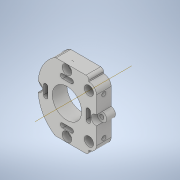
# Autodesk Inventor part: 20_Cube_Insert_Kinematic_VCAmount_Base_Thorlabs_Cage_smaller
Saved by Autodesk Inventor 2022.3 (Build 263350000, 350)
## iProperties
Created: 2019-07-01
Part Number: 20_Cube_Insert_Kinematic_VCAmount_Base_Thorlabs_Cage_smaller
Material: Generic
Document SubType Name: Modeling
Designer: diederichbenedict
Density: 1 g/cm^3
Appearance: Default
Author: diederichbenedict
Autodesk Inventor part; units mm, degrees
ref_plane "YZ Plane" through (0, 0, 0) normal (1, 0, 0) x (0, 1, 0)
ref_plane "Work Plane1" through (0, 0, 10) normal (0, 0, 1) x (1, 0, 0)
sketch "Sketch1" plane through (0, 0, 10) normal (0, 0, 1) x (1, 0, 0)
  line L0 (-4.0299, -0.3538) -> (-2.2322, 1.4439) construction
  arc A0 (-1.4439, 2.2322) -> (-2.2322, 1.4439) centre (-0.9299, 0.9299) ccw construction
  line L1 (-1.4439, 2.2322) -> (0.3538, 4.0299) construction
  line L2 (-37.8299, 42.8299) -> (-37.8299, 37.8299) construction
  line L3 (-37.8299, 37.8299) -> (-42.9208, 37.8299) construction
  line L4 (-37.8299, 42.2137) -> (-37.8299, 45.8299) construction
  line L5 (-37.8299, 45.8299) -> (-4.0299, 45.8299) construction
  line L6 (-4.0299, 45.8299) -> (-4.0299, 42.2137) construction
  line L7 (-4.0299, 4.0299) -> (0.3538, 4.0299) projected
  circle A1 centre (-20.9299, 20.9299) radius 17.5 projected
  line L8 (-20.9299, 58.9723) -> (17.1124, 20.9299) construction
  line L9 (17.1124, 20.9299) -> (-20.9299, -17.1124) construction
  line L10 (-20.9299, -17.1124) -> (-58.9723, 20.9299) construction
  line L11 (-58.9723, 20.9299) -> (-20.9299, 58.9723) construction
  line L12 (-20.9299, 58.9723) -> (-20.9299, -17.1124) construction
  line L13 (17.1124, 20.9299) -> (-58.9723, 20.9299) construction
  line L14 (-20.9299, 58.9723) -> (32.8701, 58.9723) construction
  line L15 (-43.4299, 43.4299) -> (1.5701, 43.4299) construction
  line L16 (1.5701, 43.4299) -> (1.5701, -1.5701) construction
  line L17 (1.5701, -1.5701) -> (-43.4299, -1.5701) construction
  line L18 (-43.4299, -1.5701) -> (-43.4299, 43.4299) construction
  line L19 (-43.4299, 43.4299) -> (1.5701, -1.5701) construction
  line L20 (1.5701, 43.4299) -> (-43.4299, -1.5701) construction
  line L21 (-43.4299, 5.3876) -> (-43.4299, 36.4723)
  line L22 (-43.4299, 36.4723) -> (-36.4723, 43.4299)
  line L23 (-36.4723, 43.4299) -> (-5.3876, 43.4299)
  line L24 (-5.3876, 43.4299) -> (1.5701, 36.4723)
  line L25 (1.5701, 36.4723) -> (1.5701, 5.3876)
  line L26 (1.5701, 5.3876) -> (-5.3876, -1.5701)
  line L27 (-5.3876, -1.5701) -> (-36.4723, -1.5701)
  line L28 (-36.4723, -1.5701) -> (-43.4299, 5.3876)
  line L29 (-4.0299, 42.2137) -> (-37.8299, 42.2137) projected
  line L30 (-4.0299, -0.3538) -> (-4.0299, 4.0299) projected
  point P0 (-37.8299, 4.0299)
  point P1 (-20.9299, 20.9299)
  dimension "d18" = 53.8
  dimension "d19" = 45
  dimension "d20" = 53.8
  dimension "d21" = 45
  dimension "d22" = 45
  constraints: 42 end point, 15 point on line, 5 midpoint, 4 parallel, 3 perpendicular, 2 horizontal, 1 equal length
  measures "d18" distance of L8.start L8.end
  measures "d19" angle of L8 L14
  measures "d20" distance of L8.end L9.end
  measures "d21" distance of L16.end L17.end
  measures "d22" distance of L15.end L16.end
extrude "Extrusion1" add sketch "Sketch1" along normal blind 10 contours L30 L26 L27 L28 L21 L22 L29 L24 L25 L7 | L7 L26 L30 | L29 L22 L23 L24 | A1
ref_plane "Work Plane2" through (-40.9959, 0.8639, 22.2359) normal (0, 0, 1) x (1, 0, 0)
sketch "Sketch3" plane through (0, 0, 10) normal (0, 0, -1) x (-1, 0, 0)
  line L0 (37.8299, -0.4701) -> (37.8299, 4.0299) construction
  line L1 (4.0299, 4.0299) -> (4.0299, -0.4701) construction
  line L2 (37.8299, -0.4701) -> (37.8299, 1.1886) construction
  line L3 (4.0299, -3.9701) -> (4.0299, -0.3538) construction
  line L4 (45.8299, 4.0299) -> (42.2137, 4.0299) construction
  line L5 (-0.3538, 4.0299) -> (-3.9701, 4.0299) construction
  line L6 (-3.9701, 37.8299) -> (-0.3538, 37.8299) construction
  line L7 (4.0299, 42.2137) -> (4.0299, 45.8299) construction
  line L8 (37.8299, 45.8299) -> (37.8299, 42.2137) construction
  line L9 (42.2137, 37.8299) -> (45.8299, 37.8299) construction
  line L10 (40.4657, 37.7299) -> (45.8299, 37.7299)
  line L11 (45.8299, 37.7299) -> (45.8299, 4.1299)
  line L12 (45.8299, 4.1299) -> (40.4657, 4.1299)
  line L13 (40.4657, 4.1299) -> (40.4657, 37.7299)
  line L14 (37.7299, 2.4952) -> (4.1299, 2.4952)
  line L15 (4.1299, 2.4952) -> (4.1299, -3.9701)
  line L16 (4.1299, -3.9701) -> (37.7299, -3.9701)
  line L17 (37.7299, -3.9701) -> (37.7299, 2.4952)
  line L18 (1.8946, 4.1299) -> (-3.9701, 4.1299)
  line L19 (-3.9701, 4.1299) -> (-3.9701, 37.7299)
  line L20 (-3.9701, 37.7299) -> (1.8946, 37.7299)
  line L21 (1.8946, 37.7299) -> (1.8946, 4.1299)
  line L22 (4.1299, 40.7326) -> (37.7299, 40.7326)
  line L23 (37.7299, 40.7326) -> (37.7299, 45.8299)
  line L24 (37.7299, 45.8299) -> (4.1299, 45.8299)
  line L25 (4.1299, 45.8299) -> (4.1299, 40.7326)
  point P0 (0, 0)
  dimension "d23" = 0.1
  dimension "d24" = 0.1
  dimension "d25" = 0.1
  dimension "d26" = 0.1
  dimension "d27" = 0.1
  constraints: 32 end point, 8 parallel, 4 horizontal, 4 perpendicular, 3 point on line
  measures "d23" distance between parallel lines of L8 L23
  measures "d24" distance between parallel lines of L7 L25
  measures "d25" distance between parallel lines of L6 L20
  measures "d26" distance between parallel lines of L5 L18
  measures "d27" distance between parallel lines of L1 L15
extrude "Extrusion3" add sketch "Sketch3" against normal up to surface (10 mm away)
sketch "Sketch4" plane through (0, 0, 20) normal (0, 0, 1) x (1, 0, 0)
  line L0 (3.9701, 4.1299) -> (0.3124, 4.1299) projected
  line L1 (3.9701, 37.7299) -> (3.9701, 4.1299) projected
  line L2 (0.3124, 37.7299) -> (3.9701, 37.7299) projected
  line L3 (0.3124, 37.7299) -> (-4.1299, 42.1723) projected
  line L4 (-4.1299, 45.8299) -> (-4.1299, 42.1723) projected
  line L5 (-37.7299, 45.8299) -> (-4.1299, 45.8299) projected
  line L6 (-37.7299, 42.1723) -> (-37.7299, 45.8299) projected
  line L7 (-37.7299, 42.1723) -> (-42.1723, 37.7299) projected
  line L8 (-45.8299, 37.7299) -> (-42.1723, 37.7299) projected
  line L9 (-45.8299, 4.1299) -> (-45.8299, 37.7299) projected
  line L10 (-42.1723, 4.1299) -> (-45.8299, 4.1299) projected
  line L11 (-42.1723, 4.1299) -> (-37.7299, -0.3124) projected
  line L12 (-37.7299, -3.9701) -> (-37.7299, -0.3124) projected
  line L13 (-4.1299, -3.9701) -> (-37.7299, -3.9701) projected
  line L14 (-4.1299, -0.3124) -> (-4.1299, -3.9701) projected
  line L15 (-4.1299, -0.3124) -> (0.3124, 4.1299) projected
  line L16 (-3.9799, 45.9799) -> (-3.9799, 42.2344)
  line L17 (-3.9799, 42.2344) -> (0.3745, 37.8799)
  line L18 (0.3745, 37.8799) -> (4.1201, 37.8799)
  line L19 (4.1201, 37.8799) -> (4.1201, 3.9799)
  line L20 (4.1201, 3.9799) -> (0.3745, 3.9799)
  line L21 (0.3745, 3.9799) -> (-3.9799, -0.3745)
  line L22 (-3.9799, -0.3745) -> (-3.9799, -4.1201)
  line L23 (-3.9799, -4.1201) -> (-37.8799, -4.1201)
  line L24 (-37.8799, -4.1201) -> (-37.8799, -0.3745)
  line L25 (-37.8799, -0.3745) -> (-42.2344, 3.9799)
  line L26 (-42.2344, 3.9799) -> (-45.9799, 3.9799)
  line L27 (-45.9799, 3.9799) -> (-45.9799, 37.8799)
  line L28 (-45.9799, 37.8799) -> (-42.2344, 37.8799)
  line L29 (-42.2344, 37.8799) -> (-37.8799, 42.2344)
  line L30 (-37.8799, 42.2344) -> (-37.8799, 45.9799)
  line L31 (-37.8799, 45.9799) -> (-3.9799, 45.9799)
  point P0 (0, 0)
  dimension "d34" = 0.15
  constraints: 32 end point, 15 other
  measures "d34" distance between parallel lines of L5 L31
extrude "Extrusion4" add sketch "Sketch4" against normal up to surface (10 mm away)
sketch "Sketch8" plane through (0, 0, 20) normal (0, 0, 1) x (1, 0, 0)
  circle A0 centre (-20.9299, 20.9299) radius 10
  line L0 (4.1201, 37.8799) -> (4.1201, 3.9799) projected
  line L1 (-37.8799, 45.9799) -> (-3.9799, 45.9799) projected
  point P0 (0, 0)
  point P1 (4.1201, 20.9299)
  point P2 (-20.9299, 45.9799)
  dimension "d61" = 20
  constraints: 2 midpoint, 1 centre point, 1 horizontal alignment, 1 vertical alignment
  measures "d61" diameter of A0
ref_plane "Work Plane3" through (-40.0572, 1.8027, 20) normal (-0.7071, 0.7071, 0) x (0.7071, 0.7071, 0)
sketch "Sketch5" plane through (0, 0, 20) normal (0, 0, 1) x (1, 0, 0)
  circle A0 centre (-20.9299, 20.9299) radius 29.7458 construction
  line L0 (4.1201, 37.8799) -> (4.1201, 3.9799) projected
  line L1 (-37.8799, 45.9799) -> (-3.9799, 45.9799) projected
  line L2 (-34.9299, 6.9299) -> (-6.9299, 6.9299) construction
  line L3 (-6.9299, 6.9299) -> (-6.9299, 34.9299) construction
  line L4 (-6.9299, 34.9299) -> (-34.9299, 34.9299) construction
  line L5 (-34.9299, 34.9299) -> (-34.9299, 6.9299) construction
  line L6 (-34.9299, 6.9299) -> (-6.9299, 34.9299) construction
  line L7 (-6.9299, 6.9299) -> (-34.9299, 34.9299) construction
  line L8 (-40.7289, 20.9299) -> (-20.9299, 40.7289)
  line L9 (-20.9299, 40.7289) -> (-1.1309, 20.9299)
  line L10 (-1.1309, 20.9299) -> (-20.9299, 1.1309)
  line L11 (-20.9299, 1.1309) -> (-40.7289, 20.9299)
  line L12 (-40.7289, 20.9299) -> (-1.1309, 20.9299) construction
  line L13 (-20.9299, 40.7289) -> (-20.9299, 1.1309) construction
  line L14 (-3.9799, -4.1201) -> (-37.8799, -4.1201) construction
  point P0 (0, 0)
  point P1 (4.1201, 20.9299)
  point P2 (-20.9299, 45.9799)
  point P3 (0, 0)
  point P4 (-20.9299, 20.9299)
  point P5 (-20.9299, 20.9299)
  point P6 (-20.9299, 45.9799)
  point P7 (-20.9299, -4.1201)
  point P8 (4.1201, 20.9299)
  dimension "d37" = 28
  dimension "d38" = 28
  dimension "d41" = 28
  dimension "d42" = 28
  constraints: 24 end point, 8 midpoint, 4 coincident, 4 parallel, 3 vertical alignment, 2 horizontal alignment, 2 perpendicular, 1 centre point, 1 horizontal
  measures "d37" distance of L4.end L3.end
  measures "d38" distance of L3.end L2.end
  measures "d41" distance of L10.end L8.start
  measures "d42" distance of L8.start L8.end
hole "Hole1" at (-20.9299, 40.7289, 20) at (-1.1309, 20.9299, 20) at (-20.9299, 1.1309, 20) at (-40.7289, 20.9299, 20) direction (0, 0, -1) diameter 2.85 end through all counterbore diameter 6.5 counterbore depth 4
sketch "Sketch6" plane through (0, 0, 20) normal (0, 0, 1) x (1, 0, 0)
  circle A0 centre (-1.1311, 20.9299) radius 3.25
  line L0 (-17.9299, 6.3799) -> (-23.9299, 6.3799) construction
  line L1 (-17.9299, 7.8799) -> (-23.9299, 7.8799)
  line L2 (-23.9299, 4.8799) -> (-17.9299, 4.8799)
  arc A1 (-17.9299, 4.8799) -> (-16.4299, 6.3799) centre (-17.9299, 6.3799) ccw
  arc A2 (-23.9299, 7.8799) -> (-25.4299, 6.3799) centre (-23.9299, 6.3799) ccw
  circle A3 centre (-20.9299, 40.7289) radius 3.25 projected
  line L3 (-3.9799, 45.9799) -> (-3.9799, 42.2344) projected
  line L4 (-37.8799, 45.9799) -> (-3.9799, 45.9799) projected
  line L5 (-37.8799, 42.2344) -> (-37.8799, 45.9799) projected
  line L6 (-42.2344, 37.8799) -> (-37.8799, 42.2344) projected
  line L7 (-45.9799, 37.8799) -> (-42.2344, 37.8799) projected
  line L8 (-45.9799, 3.9799) -> (-45.9799, 37.8799) projected
  line L9 (-42.2344, 3.9799) -> (-45.9799, 3.9799) projected
  line L10 (-37.8799, -0.3745) -> (-42.2344, 3.9799) projected
  line L11 (-37.8799, -4.1201) -> (-37.8799, -0.3745) projected
  line L12 (-3.9799, -4.1201) -> (-37.8799, -4.1201) projected
  line L13 (-3.9799, -0.3745) -> (-3.9799, -4.1201) projected
  line L14 (0.3745, 3.9799) -> (-3.9799, -0.3745) projected
  line L15 (4.1201, 3.9799) -> (0.3745, 3.9799) projected
  line L16 (4.1201, 37.8799) -> (4.1201, 3.9799) projected
  line L17 (0.3745, 37.8799) -> (4.1201, 37.8799) projected
  line L18 (-3.9799, 42.2344) -> (0.3745, 37.8799) projected
  circle A4 centre (-20.9299, 40.7289) radius 3.25 projected
  line L19 (-3.9799, 45.9799) -> (-3.9799, 42.2344) projected
  line L20 (-37.8799, 45.9799) -> (-3.9799, 45.9799) projected
  line L21 (-37.8799, 42.2344) -> (-37.8799, 45.9799) projected
  line L22 (-42.2344, 37.8799) -> (-37.8799, 42.2344) projected
  line L23 (-45.9799, 37.8799) -> (-42.2344, 37.8799) projected
  line L24 (-45.9799, 3.9799) -> (-45.9799, 37.8799) projected
  line L25 (-42.2344, 3.9799) -> (-45.9799, 3.9799) projected
  line L26 (-37.8799, -0.3745) -> (-42.2344, 3.9799) projected
  line L27 (-37.8799, -4.1201) -> (-37.8799, -0.3745) projected
  line L28 (-3.9799, -4.1201) -> (-37.8799, -4.1201) projected
  line L29 (-3.9799, -0.3745) -> (-3.9799, -4.1201) projected
  line L30 (0.3745, 3.9799) -> (-3.9799, -0.3745) projected
  line L31 (4.1201, 3.9799) -> (0.3745, 3.9799) projected
  line L32 (4.1201, 37.8799) -> (4.1201, 3.9799) projected
  line L33 (0.3745, 37.8799) -> (4.1201, 37.8799) projected
  line L34 (-3.9799, 42.2344) -> (0.3745, 37.8799) projected
  line L35 (-23.9299, 33.9799) -> (-17.9299, 33.9799)
  arc A5 (-23.9299, 36.9799) -> (-25.4299, 35.4799) centre (-23.9299, 35.4799) ccw
  arc A6 (-17.9299, 33.9799) -> (-16.4299, 35.4799) centre (-17.9299, 35.4799) ccw
  line L36 (-17.9299, 36.9799) -> (-23.9299, 36.9799)
  line L37 (-17.9299, 35.4799) -> (-23.9299, 35.4799) construction
  arc A7 (-7.8799, 17.9341) -> (-6.3799, 16.4341) centre (-6.3799, 17.9341) ccw
  line L38 (-7.8799, 23.9299) -> (-7.8799, 17.9341)
  line L39 (-6.3799, 17.9341) -> (-6.3799, 22.4299) construction
  line L40 (-4.8799, 17.9341) -> (-4.8799, 23.9299)
  circle A8 centre (-20.9299, 40.7289) radius 3.25
  arc A9 (-4.8799, 23.9299) -> (-6.3799, 25.4299) centre (-6.3799, 23.9299) ccw
  line L41 (-45.9799, 3.9799) -> (-45.9799, 37.8799) projected
  circle A10 centre (-40.7289, 20.9299) radius 3.25 projected
  circle A11 centre (-40.7289, 20.9299) radius 1.425 projected
  line L42 (4.1201, 37.8799) -> (4.1201, 3.9799) projected
  circle A12 centre (-20.9299, 1.1309) radius 3.25 projected
  circle A13 centre (-20.9299, 1.1309) radius 1.425 projected
  line L43 (-37.8799, 45.9799) -> (-3.9799, 45.9799) projected
  line L44 (-3.9799, -4.1201) -> (-37.8799, -4.1201) projected
  arc A14 (-6.3799, 16.4341) -> (-4.8799, 17.9341) centre (-6.3799, 17.9341) ccw
  arc A15 (-6.3799, 25.4299) -> (-7.8799, 23.9299) centre (-6.3799, 23.9299) ccw
  line L45 (-6.3799, 22.4299) -> (-6.3799, 23.9299) construction
  arc A16 (-16.4299, 35.4799) -> (-17.9299, 36.9799) centre (-17.9299, 35.4799) ccw
  arc A17 (-25.4299, 35.4799) -> (-23.9299, 33.9799) centre (-23.9299, 35.4799) ccw
  arc A18 (-16.4299, 6.3799) -> (-17.9299, 7.8799) centre (-17.9299, 6.3799) ccw
  arc A19 (-25.4299, 6.3799) -> (-23.9299, 4.8799) centre (-23.9299, 6.3799) ccw
  circle A20 centre (-40.7289, 20.9299) radius 3.25
  arc A21 (-36.8215, 17.9341) -> (-35.3215, 16.4341) centre (-35.3215, 17.9341) ccw
  line L46 (-36.8215, 23.9257) -> (-36.8215, 17.9341)
  line L47 (-35.3215, 23.9257) -> (-35.3215, 19.4341) construction
  line L48 (-33.8215, 17.9341) -> (-33.8215, 23.9257)
  arc A22 (-33.8215, 23.9257) -> (-35.3215, 25.4257) centre (-35.3215, 23.9257) ccw
  arc A23 (-35.3215, 25.4257) -> (-36.8215, 23.9257) centre (-35.3215, 23.9257) ccw
  arc A24 (-35.3215, 16.4341) -> (-33.8215, 17.9341) centre (-35.3215, 17.9341) ccw
  line L49 (-35.3215, 19.4341) -> (-35.3215, 17.9341) construction
  point P0 (-20.9299, 6.3799)
  point P1 (-20.9299, 20.9299)
  point P2 (-20.9299, 45.9799)
  point P3 (-45.9799, 20.9299)
  point P4 (4.1201, 20.9299)
  point P5 (-40.7289, 40.7289)
  point P6 (-20.9299, 35.4799)
  point P7 (66.7709, 47.2309)
  point P8 (-45.9801, 20.9299)
  point P9 (-1.8027, 1.8027)
  point P10 (-20.9299, 7.8799)
  point P11 (-6.3799, 20.9299)
  point P12 (-20.9299, 45.9802)
  point P13 (-40.0572, 40.0572)
  point P14 (-20.9299, 36.9799)
  point P15 (-1.8027, 40.0572)
  point P16 (-4.8799, 20.932)
  point P17 (-1.8027, 40.0572)
  point P18 (-45.9801, 20.9299)
  point P19 (-40.0573, 1.8027)
  point P20 (-40.0573, 1.8027)
  point P21 (-20.9299, 45.9799)
  point P22 (4.1201, 20.9299)
  point P23 (4.1201, 20.9299)
  point P24 (-20.9299, -4.1201)
  point P25 (-35.4799, 20.9299)
  point P26 (-36.8215, 20.9299)
  dimension "d52" = 3
  dimension "d53" = 3
  dimension "d87" = 3
  dimension "d88" = 3
  dimension "d91" = 3
  dimension "d92" = 3
  dimension "d130" = 10.5
  dimension "d131" = 10.5
  dimension "d132" = 10.5
  dimension "d159" = 3
  dimension "d160" = 3
  dimension "d161" = 10.5
  dimension "d162" = 5.2489
  dimension "d163" = 5.249
  constraints: 34 end point, 34 point on circle, 32 tangent, 19 centre point, 17 midpoint, 10 point on line, 8 horizontal alignment, 8 parallel, 4 vertical alignment, 1 coincident
  measures "d52" distance of point (-20.93, 6.38) L0.end
  measures "d53" diameter of A2
  measures "d87" distance of point (-20.93, 35.48) L37.end
  measures "d88" diameter of A5
  measures "d91" distance of point (-6.38, 20.93) L45.end
  measures "d92" diameter of A9
  measures "d130" distance from line of L4 point (-20.93, 35.48)
  measures "d131" distance from line of L16 point (-6.38, 20.93)
  measures "d132" distance from line of L12 point (-20.93, 6.38)
  measures "d159" distance of point (-35.48, 20.93) L49.end
  measures "d160" diameter of A21
  measures "d161" distance from line of L8 point (-35.48, 20.93)
  measures "d162" distance of A0.centre point (-6.38, 20.93)
  measures "d163" distance of point (-35.48, 20.93) A10.centre
extrude "Extrusion5" cut sketch "Sketch6" against normal through all contours A18 A1 L2 A19 A2 L1 | A17 A5 L36 A16 A6 L35 | L38 A15 A9 L40 A14 A7 | L46 A23 A22 L48 A24 A21
extrude "Extrusion6" cut sketch "Sketch8" against normal through all
sketch "Sketch2" plane through (0, 0, 20) normal (0, 0, 1) x (1, 0, 0)
  circle A0 centre (-35.9299, 35.9299) radius 3.0099 construction
  circle A1 centre (-5.93, 35.9299) radius 3.0099 construction
  circle A2 centre (-5.93, 5.93) radius 3.0099 construction
  circle A3 centre (-35.9299, 5.93) radius 3.0099 construction
  circle A4 centre (-35.9299, 35.9299) radius 3.125 construction
  circle A5 centre (-5.93, 35.9299) radius 3.125 construction
  circle A6 centre (-5.93, 5.93) radius 3.125 construction
  circle A7 centre (-35.9299, 5.93) radius 3.125 construction
  line L0 (1.5701, 5.3876) -> (1.5701, 36.4723) projected
  line L1 (-5.3876, 43.4299) -> (-36.4723, 43.4299) projected
  line L2 (-36.4723, 43.4299) -> (-43.4299, 36.4723) projected
  line L3 (-4.8799, 23.9299) -> (-4.8799, 17.9341) projected
  line L4 (-23.9299, 7.8799) -> (-17.9299, 7.8799) projected
  line L5 (-23.9299, 36.9799) -> (-17.9299, 36.9799) projected
  circle A8 centre (-5.93, 5.93) radius 5.1
  circle A9 centre (-5.93, 35.9299) radius 5.1
  point P0 (0, 0)
  point P1 (-20.9299, 20.9299)
  point P2 (1.5701, 20.9299)
  point P3 (-20.9299, 43.4299)
  point P4 (-35.9299, 35.9299)
  point P5 (-38.1396, 38.1396)
  point P6 (-36.7387, 32.9114)
  point P7 (-32.9114, 36.7387)
  point P8 (-5.1211, 32.9114)
  point P9 (-4.0799, 33.1904)
  point P10 (-4.1189, 8.6799)
  point P11 (-9.902, 8.6799)
  dimension "d31" = 6.25
  dimension "d32" = 6.25
  dimension "d33" = 6.25
  dimension "d102" = 6.25
  dimension "d110" = 0.2412
  dimension "d140" = 10.2
  dimension "d141" = 10.2
  constraints: 6 centre point, 3 point on circle, 2 midpoint, 1 coincident, 1 horizontal alignment, 1 vertical alignment
  measures "d31" diameter of A5
  measures "d32" diameter of A6
  measures "d33" diameter of A7
  measures "d102" diameter of A4
  measures "d110" distance from line of L3 point (-5.121, 32.911)
  measures "d140" diameter of A8
  measures "d141" diameter of A9
sketch "Sketch9" plane through (4.1201, 3.9799, 20) normal (1, 0, 0) x (0, 0, -1)
  line L0 (0, 0) -> (10, 0) projected
  line L1 (0, 33.9) -> (10, 33.9) projected
  point P0 (20, -3.9799)
  point P1 (5, 4)
  point P2 (5, 0)
  point P3 (5, 29.9)
  point P4 (5, 33.9)
  dimension "d64" = 4
  dimension "d65" = 4
  constraints: 2 midpoint, 2 vertical alignment
  measures "d64" distance from line of L0 point (5, 4)
  measures "d65" distance from line of L1 point (5, 29.9)
hole "Hole2" at (4.1201, 7.9799, 15) at (4.1201, 33.8799, 15) direction (-1, 0, 0) diameter 2.9 depth 10 tip angle 118
extrude "Extrusion7" [suppressed]
sketch "Sketch10" plane through (0, 0, 20) normal (0, 0, 1) x (1, 0, 0)
  line L0 (-37.8799, 45.9799) -> (-3.9799, 45.9799) projected
  line L1 (-36.4799, 45.9799) -> (-37.0382, 45.9799)
  line L2 (-42.2344, 3.9799) -> (-45.9799, 3.9799) projected
  line L3 (-45.9799, 3.9799) -> (-42.2344, 3.9799)
  line L4 (-3.9799, 45.9799) -> (-3.9799, 42.2344) projected
  line L5 (-3.9799, 43.9799) -> (-5.9799, 43.9799)
  line L6 (-36.4799, 45.9799) -> (-34.1344, 45.9799)
  line L7 (-3.9799, 43.9799) -> (-3.9799, 45.9799)
  line L8 (-3.9799, -4.1201) -> (-3.9799, -2.1201)
  line L9 (-3.9799, -0.3745) -> (-3.9799, -4.1201) projected
  line L10 (-3.9799, -2.1201) -> (-5.7255, -2.1201)
  line L11 (-34.1344, 45.9799) -> (-28.9151, 45.9799)
  circle A0 centre (-5.93, 5.93) radius 3.0099 projected
  circle A1 centre (-5.93, 35.9299) radius 3.0099 projected
  arc A2 (-0.83, 5.93) -> (-5.9799, 0.8302) centre (-5.93, 5.93) ccw
  arc A3 (-3.9799, 40.6424) -> (-5.9799, 41.0297) centre (-5.93, 35.9299) ccw
  line L12 (-3.9799, 43.9799) -> (-3.9799, 40.6424)
  line L13 (-0.83, 35.9299) -> (-0.83, 24.166)
  line L14 (-3.9799, -0.3745) -> (-3.9799, 1.2175)
  line L15 (-5.9799, -2.171) -> (-5.9799, 0.8302)
  line L16 (-5.9799, 41.0297) -> (-5.9799, 43.9799)
  circle A4 centre (-1.1309, 20.9299) radius 3.25 projected
  circle A5 centre (-1.1309, 20.9299) radius 1.425 projected
  circle A6 centre (-1.1309, 20.9299) radius 3.25 projected
  line L17 (-3.9799, -4.1201) -> (-0.83, -4.1201)
  line L18 (6.2025, -4.1201) -> (6.2025, 45.9799)
  line L19 (6.2025, 45.9799) -> (4.1201, 45.9799)
  circle A7 centre (-5.93, 5.93) radius 3.1599
  circle A8 centre (-5.93, 35.9299) radius 3.1599
  arc A9 (-3.9799, 1.2175) -> (-1.2175, 3.9799) centre (-5.93, 5.93) ccw
  arc A10 (-1.2175, 3.9799) -> (-0.83, 5.93) centre (-5.93, 5.93) ccw
  line L20 (-0.83, 17.6939) -> (-0.83, 5.93)
  line L21 (-0.83, 24.166) -> (-0.83, 17.6939)
  arc A11 (-0.83, 35.9299) -> (-1.2175, 37.8799) centre (-5.93, 35.9299) ccw
  arc A12 (-5.9799, 41.0297) -> (-10.6424, 37.8799) centre (-5.93, 35.9299) ccw
  line L22 (0.3745, 3.9799) -> (-3.9799, -0.3745) projected
  line L23 (-3.9799, -0.3745) -> (-3.9799, -2.1201)
  line L24 (-3.9799, 1.2175) -> (-3.9799, -0.3745)
  line L25 (-5.9799, 41.0297) -> (-5.9799, 43.9799)
  line L26 (-3.9799, 43.9799) -> (-3.9799, 40.6424)
  line L27 (-3.9799, -0.3745) -> (-3.9799, -2.1201)
  arc A13 (-5.9799, 0.8302) -> (-3.9799, 1.2175) centre (-5.93, 5.93) ccw
  line L28 (-5.7255, -2.1201) -> (-5.9799, -2.171)
  arc A14 (-10.6424, 37.8799) -> (-0.83, 35.9299) centre (-5.93, 35.9299) ccw
  arc A15 (-1.2175, 37.8799) -> (-3.9799, 40.6424) centre (-5.93, 35.9299) ccw
  line L29 (-0.83, 45.9799) -> (-3.9799, 45.9799)
  line L30 (-5.9799, 45.9799) -> (-3.9799, 45.9799)
  line L31 (-28.9151, 45.9799) -> (-5.9799, 45.9799)
  line L32 (-37.0382, 45.9799) -> (-37.8799, 45.9799)
  line L33 (-5.9799, -4.1201) -> (-3.9799, -4.1201)
  line L34 (4.1201, 37.8799) -> (4.1201, 3.9799) projected
  line L35 (-3.9799, -4.1201) -> (-37.8799, -4.1201) projected
  line L36 (-5.9799, -4.1201) -> (-7.7255, -4.1201)
  line L37 (-37.8799, -0.3745) -> (-42.2344, 3.9799) projected
  line L38 (-37.8799, -4.1201) -> (-37.8799, -2.1201)
  line L39 (-37.8799, -0.3745) -> (-42.2344, 3.9799)
  line L40 (-42.2344, 3.9799) -> (-45.9799, 3.9799)
  line L41 (-45.9799, 3.9799) -> (-45.9799, 37.8799) projected
  line L42 (-45.9799, 3.9799) -> (-45.9799, 7.7255)
  line L43 (-42.2344, 37.8799) -> (-37.8799, 42.2344) projected
  line L44 (-45.9799, 37.8799) -> (-42.2344, 37.8799)
  line L45 (-42.2344, 37.8799) -> (-37.8799, 42.2344)
  line L46 (-37.8799, 45.9799) -> (-3.9799, 45.9799) projected
  line L47 (-37.8799, 42.2344) -> (-37.8799, 43.9799)
  line L48 (-37.8799, 43.9799) -> (-37.8799, 45.9799)
  line L49 (-45.9799, 34.1344) -> (-45.9799, 37.8799)
  line L50 (-45.9799, 7.7255) -> (-45.9799, 34.1344)
  line L51 (-37.8799, -2.1201) -> (-37.8799, -0.3745)
  line L52 (-34.1344, -4.1201) -> (-37.8799, -4.1201)
  line L53 (-7.7255, -4.1201) -> (-25.1869, -4.1201)
  line L54 (-0.83, -4.1201) -> (6.2025, -4.1201)
  line L55 (4.1201, 45.9799) -> (-0.83, 45.9799)
  line L56 (-5.9799, 43.9799) -> (-28.9151, 43.9799)
  line L57 (-5.9799, -2.171) -> (-28.9151, -2.171)
  circle A16 centre (-40.7289, 20.9299) radius 3.25 projected
  line L58 (-40.4789, 17.6896) -> (-40.4789, 24.1703)
  arc A17 (-40.4789, 17.6896) -> (-37.8799, 7.7697) centre (-15.5098, 18.931) ccw
  arc A18 (-28.9151, 43.9799) -> (-35.5096, 37.8799) centre (-15.5124, 22.8762) ccw
  arc A19 (-37.8799, 7.7697) -> (-35.5463, 3.9799) centre (-15.5098, 18.931) ccw
  arc A20 (-37.8799, 34.0429) -> (-40.4789, 24.1703) centre (-15.5124, 22.8762) ccw
  arc A21 (-28.995, -2.1201) -> (-28.9151, -2.171) centre (-15.5098, 18.931) ccw
  arc A22 (-35.5463, 3.9799) -> (-28.995, -2.1201) centre (-15.5098, 18.931) ccw
  arc A23 (-35.5096, 37.8799) -> (-37.8799, 34.0429) centre (-15.5124, 22.8762) ccw
  line L59 (-25.1869, -4.1201) -> (-34.1344, -4.1201)
  point P0 (0, 0)
  point P1 (-0.83, 24.166)
  dimension "d127" = 2
  dimension "d137" = 10.2
  dimension "d138" = 10.2
  dimension "d139" = 2
  dimension "d142" = 0.15
  dimension "d143" = 0.15
  dimension "d147" = 6.0198
  dimension "d155" = 46.151
  dimension "d157" = 25
  dimension "d158" = 25
  constraints: 99 end point, 37 point on circle, 24 point on line, 18 centre point, 15 perpendicular, 13 collinear, 12 parallel, 10 horizontal, 6 tangent, 4 vertical, 1 coincident
  measures "d127" distance between parallel lines of L0 L5
  measures "d137" diameter of A2
  measures "d138" diameter of A3
  measures "d139" distance between parallel lines of L15 L9
  measures "d142" radial gap between concentric circles of A0 A7
  measures "d143" radial gap between concentric circles of A1 A8
  measures "d147" diameter of A1
  measures "d155" distance between parallel lines of L56 L57
  measures "d157" radius of A17
  measures "d158" radius of A18
extrude "Extrusion8" cut sketch "Sketch10" against normal through all contours L0 L4 L5 L56 A18 A23 A20 A16 A17 A19 A22 A21 L57 L28 L10 L8 L33 L35 L38 L51 L37 L2 L41 L44 L43 L47 L48 | L29 L55 L19 L18 L54 L17 L8 L9 L14 A9 A10 L20 A4 L13 A11 A15 L12 L4 | L4 L12 A3 L16 L5 | L10 L28 L15 A13 L14 L9 | A0 | A1 | A7 | A8
fillet "Fillet1" radius 2 4 edges at (-5.9799, 43.9799, 15) (-5.9799, -2.171, 15) (-28.9151, -2.171, 15) (-28.9151, 43.9799, 15)
equation "\"d42\" = d41"
equation "\"d65\" = d64"
body "Solid1"
